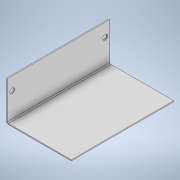
# Autodesk Inventor part: soporte de drive ws55
Saved by Autodesk Inventor 2022 (Build 260153000, 153)
## iProperties
Created: 2021-10-03
Part Number: soporte de drive ws55
Material: Genérico
Document SubType Name: Sheet Metal
Designer: andre
Density: 1 g/cm^3
Sheet Metal Rule: Por defecto
Appearance: Valor por defecto
Author: andre
Autodesk Inventor part; units mm, degrees
ref_plane "YZ Plane" through (0, 0, 0) normal (1, 0, 0) x (0, 1, 0)
ref_plane "XZ Plane" through (0, 0, 0) normal (0, 1, 0) x (-1, 0, 0)
ref_plane "XY Plane" through (0, 0, 0) normal (0, 0, 1) x (1, 0, 0)
sketch "Boceto1" plane through (0, 0, 0) normal (0, 1, 0) x (-1, 0, 0)
  line L0 (48, 48) -> (-48, 48)
  line L1 (-48, 48) -> (-48, -48)
  line L2 (-48, -48) -> (48, -48)
  line L3 (48, -48) -> (48, 48)
  line L4 (48, 48) -> (-48, -48) construction
  line L5 (-48, 48) -> (48, -48) construction
  line L6 (12, 48) -> (12, -48)
  circle A0 centre (24, 43.5) radius 2.25
  point P0 (0, 0)
  point P1 (0, 0)
  point P2 (0, 0)
  dimension "d0" = 96
  dimension "d1" = 96
  dimension "d3" = 60
  dimension "d24" = 4.5
  dimension "d25" = 12
  dimension "d26" = 4.5
  measures "d0" distance of L2.end L0.start
  measures "d1" distance of L1.end L2.end
  measures "d3" distance between parallel lines of L1 L6
  measures "d24" diameter of A0
  measures "d25" distance from line of L6 A0.centre
  measures "d26" distance from line of A0.centre L0
extrude "Placa1" add sketch "Boceto1" along normal blind 1 contours L3 L2 L6 L0 | L6 L2 L1 L0 | A0
sketch "Boceto4" plane through (0, 1, 0) normal (0, 1, 0) x (1, 0, 0)
  line L0 (-48, -48) -> (48, -48) projected
  line L1 (-12, -48) -> (-12, 48)
  line L2 (48, 48) -> (-48, 48) projected
  line L3 (48, 48) -> (48, -48) projected
  circle A0 centre (-24, -43.5) radius 2.25
  circle A1 centre (-24, 43.5) radius 2.25
  point P0 (0, 0)
  dimension "d4" = 60
  dimension "d11" = 4.5
  dimension "d12" = 12
  dimension "d13" = 4.5
  dimension "d14" = 4.5
  dimension "d15" = 12
  dimension "d16" = 4.5
  constraints: 2 centre point, 2 end point, 2 point on line, 1 vertical
  measures "d4" distance between parallel lines of L1 L3
  measures "d11" diameter of A0
  measures "d12" distance from line of L1 A0.centre
  measures "d13" distance from line of A0.centre L0
  measures "d14" diameter of A1
  measures "d15" distance from line of L1 A1.centre
  measures "d16" distance from line of L2 A1.centre
fold "Pliegue1" angle 90 bend radius 1 thickness 1 k factor 0.44 line from (-12, 1, 48) to (-12, 1, -48) line at bend centre moving side (-1, 0, 0) folds toward (0, 1, 0)
sketch "Boceto7" plane through (-11.869, 2, -48) normal (1, 0, 0) x (0, 0, -1)
  line L0 (-96, 34.869) -> (0, 34.869) projected
  line L1 (-96, 0) -> (-96, 34.869) projected
  point P0 (-48, -2)
  point P1 (-91.5, 22.869)
  dimension "d36" = 12
  dimension "d37" = 4.5
  measures "d36" distance from line of L0 point (-91.5, 22.869)
  measures "d37" distance from line of L1 point (-91.5, 22.869)
hole "Agujero3" at (-11.869, 24.869, 43.5) direction (-1, 0, 0) diameter 4.5 end through all
sketch "Boceto8" plane through (-11.869, 2, -48) normal (1, 0, 0) x (0, 0, -1)
  line L0 (-96, 34.869) -> (0, 34.869) projected
  line L1 (0, 34.869) -> (0, 0) projected
  point P0 (-48, -2)
  point P1 (-4.5, 22.869)
  dimension "d45" = 12
  dimension "d46" = 4.5
  measures "d45" distance from line of L0 point (-4.5, 22.869)
  measures "d46" distance from line of L1 point (-4.5, 22.869)
hole "Agujero4" at (-11.869, 24.869, -43.5) direction (-1, 0, 0) diameter 4.5 end through all
equation "\"d2\" = Thickness"
equation "\"d5\" = BendReliefWidth"
equation "\"d6\" = BendReliefDepth"
equation "\"d7\" = MinimumRemnant"
equation "\"d8\" = TransitionRadius"
equation "\"d10\" = BendRadius"
equation "\"BendRadius\" = Thickness"
equation "\"BendReliefWidth\" = Thickness"
equation "\"BendReliefDepth\" = 0.5 * Thickness"
equation "\"CornerReliefSize\" = 4 * Thickness"
equation "\"MinimumRemnant\" = 2 * Thickness"
equation "\"TransitionRadius\" = BendRadius"
equation "\"JacobiRadiusSize\" = BendRadius"
equation "\"GapSize\" = Thickness"
equation "\"Thickness\" = 1"
